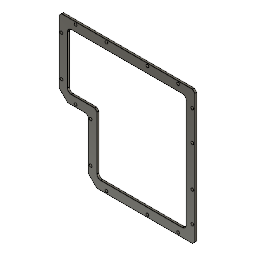
1006349-exact-GASKET, RETAINED (Autodesk Fusion 360 design; units mm, degrees)
Autodesk Fusion 360 part; units mm, degrees
note: some values were not read from the file. Set by a fixed rule: the direction of a hole.
sketch "Front" plane through (0, 0, 0) normal (0, 1, 0) x (1, 0, 0) in component "1006349"
  line L0 (-57.8768, -199.5135) -> (216.2733, -199.5135) construction
  line L1 (-57.6388, 3.5595) -> (225.0785, 3.5595) construction
  line L2 (7.3291, 79.7924) -> (7.3291, -206.2565) construction
  line L3 (213.5386, 80.0304) -> (213.5386, -202.9248) construction
  line L4 (-45.264, -185.7975) -> (221.5088, -185.7975) construction
  line L5 (-43.8142, -9.9025) -> (216.9872, -9.9025) construction
  line L6 (20.1798, 68.3695) -> (20.1798, -205.3046) construction
  line L7 (-33.6031, -100.5805) -> (90.6212, -100.5805) construction
  line L8 (-21.4662, -86.8645) -> (74.9147, -86.8645) construction
  line L9 (51.7406, 52.901) -> (51.7406, -104.1642) construction
  line L10 (64.9486, 43.6199) -> (64.9486, -104.4021) construction
  line L11 (61.3164, 31.245) -> (61.3164, -104.4021) construction
  line L12 (204.2676, 28.1453) -> (204.2676, -293.7347) construction
  line L13 (301.4692, -174.3675) -> (-2.19, -174.3675) construction
  line L14 (289.3324, -128.6475) -> (193.4275, -128.6475) construction
  line L15 (188.2402, -212.6819) -> (188.2402, 15.0626) construction
  line L16 (141.5042, -224.3428) -> (141.5042, 9.827) construction
  line L17 (79.2234, -236.9556) -> (79.2234, 11.9688) construction
  line L18 (32.4366, -262.9987) -> (32.4366, -64.0809) construction
  line L19 (55.2966, -250.3288) -> (55.2966, 19.8573) construction
  line L20 (276.3559, -113.1535) -> (-0.7101, -113.1535) construction
  line L21 (251.1435, -82.9275) -> (47.1227, -82.9275) construction
  line L22 (224.557, -21.7135) -> (42.5012, -21.7135) construction
  line L23 (328.6587, -0.2505) -> (74.127, -0.2505) construction
  line L24 (326.747, -5.7115) -> (-6.8013, -5.7115) construction
  line L25 (238.6648, -67.4335) -> (193.169, -67.4335) construction
  line L26 (209.7286, -275.7982) -> (209.7286, -12.1057) construction
  line L27 (313.957, -195.7035) -> (25.5151, -195.7035) construction
  line L28 (325.8246, -190.0139) -> (-1.5489, -190.0139) construction
  line L29 (263.2084, -90.6745) -> (24.7432, -90.6745) construction
  line L30 (10.999, -276.0365) -> (10.999, -104.4195) construction
  line L31 (16.7648, -288.1351) -> (16.7648, -78.75) construction
  line L32 (7.3291, -199.5135) -> (213.5386, -199.5135)
  line L33 (213.5386, 3.5595) -> (51.7406, 3.5595)
  line L34 (51.7406, -86.8645) -> (51.7406, 3.5595)
  line L35 (51.7406, -86.8645) -> (7.3291, -86.8645)
  line L36 (7.3291, -86.8645) -> (7.3291, -199.5135)
  line L37 (213.5386, -199.5135) -> (213.5386, 3.5595)
  line L38 (20.1798, -104.5315) -> (20.1798, -100.5805)
  line L39 (200.0766, -193.5194) -> (200.0766, 68.0398) construction
  line L40 (-6.7988, -96.9737) -> (70.6703, -96.9737) construction
  line L41 (20.1798, -185.7975) -> (200.0766, -185.7975)
  line L42 (200.0766, -185.7975) -> (200.0766, -5.7115)
  line L43 (64.9486, -5.7115) -> (64.9486, -100.5805)
  line L44 (64.9486, -100.5805) -> (20.1798, -100.5805)
  line L45 (20.1798, -100.5805) -> (20.1798, -185.7975)
  line L46 (200.0766, -9.9025) -> (64.9486, -9.9025)
  point P0 (10.999, -174.3675)
  point P1 (32.4366, -195.7035)
  point P2 (79.2234, -195.7035)
  point P3 (141.5042, -195.7035)
  point P4 (188.2402, -195.7035)
  point P5 (209.7286, -174.3675)
  point P6 (209.7286, -128.6475)
  point P7 (209.7286, -67.4335)
  point P8 (209.7286, -21.7135)
  point P9 (188.2402, -0.2505)
  point P10 (141.5042, -0.2505)
  point P11 (79.2234, -0.2505)
  point P12 (55.2966, -21.7135)
  point P13 (55.2966, -82.9275)
  point P14 (32.4366, -90.6745)
  point P15 (10.999, -113.1535)
  dimension "d1" = 203.073
  dimension "d2" = 174.117
  dimension "d3" = 128.397
  dimension "d4" = 90.424
  dimension "d5" = 82.677
  dimension "d6" = 67.183
  dimension "d7" = 21.463
  dimension "d8" = 195.453
  dimension "d9" = 90.424
  dimension "d10" = 13.462
  dimension "d14" = 198.7296
  dimension "d15" = 177.292
  dimension "d16" = 154.432
  dimension "d17" = 130.5052
  dimension "d18" = 68.2244
  dimension "d19" = 21.4884
  dimension "d20" = 161.798
  dimension "d22" = 142.9512
  dimension "d26" = 175.895
  dimension "d27" = 112.903
  dimension "d28" = 184.3024
  dimension "d31" = 5.461
  dimension "d32" = 13.716
  dimension "d33" = 187.5028
  dimension "d46" = 9.652
  dimension "d48" = 13.462
  dimension "d49" = 135.128
  dimension "d50" = 91.2622
  dimension "d51" = 5.461
  constraint horizontal L0
  constraint horizontal L1
  constraint perpendicular L0 L2
  constraint vertical L3
  constraint perpendicular L3 L4
  constraint perpendicular L3 L5
  constraint perpendicular L0 L6
  constraint perpendicular L2 L7
  constraint perpendicular L2 L8
  constraint perpendicular L8 L9
  constraint perpendicular L7 L10
  constraint perpendicular L7 L11
  constraint perpendicular L0 L12
  constraint perpendicular L3 L13
  constraint perpendicular L1 L15
  constraint perpendicular L5 L16
  constraint perpendicular L1 L17
  constraint perpendicular L8 L18
  constraint perpendicular L1 L19
  constraint perpendicular L2 L20
  constraint perpendicular L9 L21
  constraint perpendicular L9 L22
  constraint perpendicular L17 L23
  constraint perpendicular L2 L24
  constraint perpendicular L22 L26
  constraint perpendicular L6 L27
  constraint perpendicular L2 L28
  constraint perpendicular L6 L29
  constraint perpendicular L7 L30
  constraint perpendicular L8 L31
  constraint coincident L0 L32.start
  constraint coincident L2 L32.start
  constraint coincident L3 L32.end
  constraint coincident L0 L32.end
  constraint coincident L3 L33.start
  constraint coincident L1 L33.start
  constraint coincident L9 L33.end
  constraint coincident L1 L33.end
  constraint coincident L8 L34.start
  constraint coincident L9 L34.start
  constraint coincident L8 L35.end
  constraint coincident L2 L35.end
  constraint coincident L30 P0
  constraint coincident L13 P0
  constraint coincident L18 P1
  constraint coincident L27 P1
  constraint coincident L17 P2
  constraint coincident L27 P2
  constraint coincident L16 P3
  constraint coincident L27 P3
  constraint coincident L15 P4
  constraint coincident L27 P4
  constraint coincident L26 P5
  constraint coincident L13 P5
  constraint coincident L14 P6
  constraint coincident L26 P6
  constraint coincident L25 P7
  constraint coincident L26 P7
  constraint coincident L22 P8
  constraint coincident L26 P8
  constraint coincident L15 P9
  constraint coincident L23 P9
  constraint coincident L16 P10
  constraint coincident L23 P10
  constraint coincident L23 P11
  constraint coincident L17 P11
  constraint coincident L22 P12
  constraint coincident L19 P12
  constraint coincident L21 P13
  constraint coincident L19 P13
  constraint coincident L18 P14
  constraint coincident L29 P14
  constraint coincident L20 P15
  constraint coincident L30 P15
  constraint coincident L6 L38.end
  constraint coincident L7 L38.end
  constraint perpendicular L28 L39
  constraint perpendicular L19 L40
  constraint coincident L6 L41.start
  constraint coincident L4 L41.start
  constraint coincident L39 L41.end
  constraint coincident L4 L41.end
  constraint coincident L24 L42.end
  constraint coincident L39 L42.end
  constraint coincident L24 L43.start
  constraint coincident L10 L43.start
  constraint coincident L10 L43.end
  constraint coincident L7 L43.end
  constraint coincident L39 L46.start
  constraint coincident L5 L46.start
  constraint coincident L43 L46.end
  constraint coincident L5 L46.end
  measures "d1" distance of L0 L1
  measures "d2" distance of L13 L23
  measures "d3" distance of L14 L23
  measures "d4" distance of L23 L29
  measures "d5" distance of L21 L23
  measures "d6" distance of L23 L25
  measures "d7" distance of L22 L23
  measures "d8" distance of L23 L27
  measures "d9" distance of L1 L8
  measures "d10" distance of L1 L5
  measures "d14" distance of L26 L30
  measures "d15" distance of L18 L26
  measures "d16" distance of L19 L26
  measures "d17" distance of L17 L26
  measures "d18" distance of L16 L26
  measures "d19" distance of L15 L26
  measures "d20" distance of L3 L9
  measures "d22" distance of L11 L12
  measures "d26" distance of L4 L5
  measures "d27" distance of L20 L23
  measures "d28" distance of L24 L28
  measures "d31" distance of L12 L26
  measures "d32" distance of L7 L8
  measures "d33" distance of L12 L31
  measures "d46" distance of L5 L23
  measures "d48" distance of L3 L39
  measures "d49" distance of L10 L39
  measures "d50" distance of L24 L40
  measures "d51" distance of L23 L24
extrude "Extrude2" add sketch "Front" along normal blind 3.175 in component "1006349"
chamfer "Chamfer3" distance 3.556 angle 45 4 edges at (213.5386, 1.5875, -3.5595) (64.9486, 1.5875, 100.5805) (7.3291, 1.5875, 199.5135) (213.5386, 1.5875, 199.5135) in component "1006349"
chamfer "Chamfer4" distance 12.7 angle 45 2 edges at (7.3291, 1.5875, 86.8645) (51.7406, 1.5875, -3.5595) in component "1006349"
fillet "Fillet2" radius 5.5372 6 edges at (20.1798, 1.5875, 185.7975) (20.1798, 1.5875, 100.5805) (64.9486, 1.5875, 9.9025) (200.0766, 1.5875, 9.9025) (200.0766, 1.5875, 185.7975) (51.7406, 1.5875, 86.8645) in component "1006349"
hole "Hole2" at (32.4366, 0, 195.7035) at (79.2234, 0, 195.7035) at (141.5042, 0, 195.7035) at (188.2402, 0, 195.7035) at (10.999, 0, 174.3675) at (10.999, 0, 113.1535) at (32.4366, 0, 90.6745) at (209.7286, 0, 174.3675) at (209.7286, 0, 128.6475) at (209.7286, 0, 67.4335) at (209.7286, 0, 21.7135) at (188.2402, 0, 0.2505) at (141.5042, 0, 0.2505) at (79.2234, 0, 0.2505) at (55.2966, 0, 21.7135) at (55.2966, 0, 82.9275) direction (0, 1, 0) diameter 4.0894 end through all in component "1006349"
component "1006349" placed x (1, 0, 0) y (0, 1, 0) z (0, 0, 1) at (0, 0, 0)
